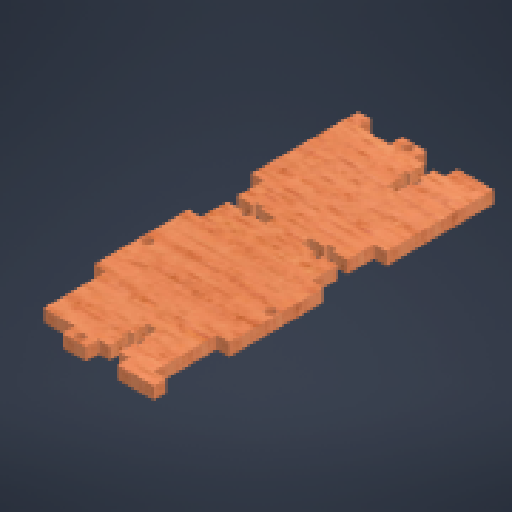
# Autodesk Inventor part: FloorButtonHolder_Top_V1
Saved by Autodesk Inventor 2024.1 (Build 281209000, 209)
## iProperties
Created: 2023-05-20
Part Number: FloorButtonHolder_Top_V1
Material: MDF Medium Density Fiberboard
Document SubType Name: Modeling
Designer: jaege
Density: 0.8 g/cm^3
Appearance: Red Oak - Natural Low Gloss
Author: jaege
Autodesk Inventor part; units mm, degrees
ref_plane "YZ Plane" through (0, 0, 0) normal (1, 0, 0) x (0, 1, 0)
ref_plane "XZ Plane" through (0, 0, 0) normal (0, 1, 0) x (-1, 0, 0)
ref_plane "XY Plane" through (0, 0, 0) normal (0, 0, 1) x (1, 0, 0)
sketch "Sketch1" plane through (0, 0, 0) normal (0, 1, 0) x (-1, 0, 0)
  line L0 (-17.5, 50) -> (17.5, 50)
  line L1 (17.5, 50) -> (17.5, -50)
  line L2 (17.5, -50) -> (-17.5, -50)
  line L3 (-17.5, -50) -> (-17.5, 50)
  line L4 (-17.5, 50) -> (17.5, -50) construction
  line L5 (17.5, 50) -> (-17.5, -50) construction
  line L6 (7.5, 50) -> (0, 50)
  line L7 (0, 50) -> (0, 54)
  line L8 (0, 54) -> (7.5, 54)
  line L9 (7.5, 54) -> (7.5, 50)
  line L10 (-10, 50) -> (-21.5, 50)
  line L11 (-21.5, 50) -> (-21.5, 54)
  line L12 (-21.5, 54) -> (-10, 54)
  line L13 (-10, 54) -> (-10, 50)
  line L14 (17.5, 30) -> (21.5, 30)
  line L15 (21.5, 30) -> (21.5, 0)
  line L16 (21.5, 0) -> (17.5, 0)
  line L17 (17.5, 0) -> (17.5, 30)
  line L18 (17.5, -20) -> (21.5, -20)
  line L19 (21.5, -20) -> (21.5, -54)
  line L20 (21.5, -54) -> (17.5, -54)
  line L21 (17.5, -54) -> (17.5, -20)
  line L22 (7.5, -50) -> (0, -50)
  line L23 (0, -50) -> (0, -54)
  line L24 (0, -54) -> (7.5, -54)
  line L25 (7.5, -54) -> (7.5, -50)
  line L26 (-10, -50) -> (-21.5, -50)
  line L27 (-21.5, -50) -> (-21.5, -54)
  line L28 (-21.5, -54) -> (-10, -54)
  line L29 (-10, -54) -> (-10, -50)
  line L30 (-17.5, 30) -> (-21.5, 30)
  line L31 (-21.5, 30) -> (-21.5, 0)
  line L32 (-21.5, 0) -> (-17.5, 0)
  line L33 (-17.5, 0) -> (-17.5, 30)
  line L34 (-17.5, -50) -> (-21.5, -50)
  line L35 (-21.5, -50) -> (-21.5, -20)
  line L36 (-21.5, -20) -> (-17.5, -20)
  line L37 (-17.5, -20) -> (-17.5, -50)
  point P0 (0, 0)
  point P1 (17.5, 0)
  point P2 (-17.5, 0)
  point P3 (-17.5, -20)
  point P4 (0, -50)
  point P5 (17.5, -50)
  dimension "d0" = 35
  dimension "d2" = 7.5
  dimension "d3" = 4
  dimension "d4" = 11.5
  dimension "d5" = 4
  dimension "d6" = 10
  dimension "d7" = 10
  dimension "d8" = 4
  dimension "d9" = 30
  dimension "d10" = 4
  dimension "d11" = 34
  dimension "d12" = 20
  dimension "d13" = 20
  dimension "d14" = 7.5
  dimension "d15" = 4
  dimension "d16" = 11.5
  dimension "d17" = 4
  dimension "d18" = 10
  dimension "d19" = 10
  dimension "d20" = 4
  dimension "d21" = 30
  dimension "d22" = 20
  dimension "d23" = 4
  dimension "d24" = 30
  dimension "d27" = 4
  constraints: 76 end point, 18 parallel, 9 horizontal, 9 perpendicular, 7 point on line, 2 midpoint
  measures "d0" distance of L1.end L2.end
  measures "d2" distance of L7.end L8.end
  measures "d3" distance of L6.end L7.end
  measures "d4" distance of L11.end L12.end
  measures "d5" distance of L10.end L11.end
  measures "d6" distance between parallel lines of L9 L1
  measures "d7" distance between parallel lines of L13 L7
  measures "d8" distance of L15.end L16.end
  measures "d9" distance of L14.end L15.end
  measures "d10" distance of L19.end L20.end
  measures "d11" distance of L18.end L19.end
  measures "d12" distance between parallel lines of L16 L18
  measures "d13" distance between parallel lines of L0 L14
  measures "d14" distance of L24.end L23.end
  measures "d15" distance of L23.end L22.end
  measures "d16" distance of L28.end L27.end
  measures "d17" distance of L27.end L26.end
  measures "d18" distance between parallel lines of L25 L21
  measures "d19" distance between parallel lines of L29 L23
  measures "d20" distance of L32.end L31.end
  measures "d21" distance of L31.end L30.end
  measures "d22" distance between parallel lines of L10 L30
  measures "d23" distance of L35.end L36.end
  measures "d24" distance of L34.end L35.end
  measures "d27" distance between parallel lines of L2 L20
extrude "Extrusion1" add sketch "Sketch1" along normal blind 4
sketch "Sketch3" plane through (0, 4, 0) normal (0, 1, 0) x (1, 0, 0)
  line L0 (17.5, 11.5) -> (5.5, 11.5)
  line L1 (5.5, 11.5) -> (5.5, 8.5)
  line L2 (5.5, 8.5) -> (17.5, 8.5)
  line L3 (17.5, 8.5) -> (17.5, 11.5)
  line L4 (10.3, 7.3) -> (12.7, 7.3)
  line L5 (12.7, 7.3) -> (12.7, 12.7)
  line L6 (12.7, 12.7) -> (10.3, 12.7)
  line L7 (10.3, 12.7) -> (10.3, 7.3)
  line L8 (17.5, 0) -> (17.5, 20) projected
  line L9 (10, -50) -> (0, -50) projected
  line L10 (3.5, -38) -> (6.5, -38)
  line L11 (6.5, -38) -> (6.5, -50)
  line L12 (6.5, -50) -> (3.5, -50)
  line L13 (3.5, -50) -> (3.5, -38)
  line L14 (2.3, -45.2) -> (7.7, -45.2)
  line L15 (7.7, -45.2) -> (7.7, -42.8)
  line L16 (7.7, -42.8) -> (2.3, -42.8)
  line L17 (2.3, -42.8) -> (2.3, -45.2)
  line L18 (-17.5, 11.5) -> (-5.5, 11.5)
  line L19 (-5.5, 11.5) -> (-5.5, 8.5)
  line L20 (-5.5, 8.5) -> (-17.5, 8.5)
  line L21 (-17.5, 8.5) -> (-17.5, 11.5)
  line L22 (-12.7, 7.3) -> (-10.3, 7.3)
  line L23 (-10.3, 7.3) -> (-10.3, 12.7)
  line L24 (-10.3, 12.7) -> (-12.7, 12.7)
  line L25 (-12.7, 12.7) -> (-12.7, 7.3)
  line L26 (0, -50) -> (10, -50) projected
  line L27 (-17.5, 20) -> (-17.5, 0) projected
  line L28 (3.5, 50) -> (6.5, 50)
  line L29 (6.5, 50) -> (6.5, 38)
  line L30 (6.5, 38) -> (3.5, 38)
  line L31 (3.5, 38) -> (3.5, 50)
  line L32 (10, 50) -> (0, 50) projected
  line L33 (2.3, 42.8) -> (7.7, 42.8)
  line L34 (7.7, 42.8) -> (7.7, 45.2)
  line L35 (7.7, 45.2) -> (2.3, 45.2)
  line L36 (2.3, 45.2) -> (2.3, 42.8)
  line L37 (10, 50) -> (0, 50) projected
  circle A0 centre (-19.5, -15) radius 1.5
  line L38 (0, 54) -> (-7.5, 54) projected
  line L39 (-7.5, 54) -> (0, 50) construction
  line L40 (-7.5, -54) -> (0, -54) projected
  line L41 (-7.5, -54) -> (0, -50) construction
  line L42 (-17.5, 0) -> (-21.5, 0) projected
  line L43 (-21.5, -30) -> (-17.5, 0) construction
  line L44 (21.5, 0) -> (17.5, 0) projected
  line L45 (17.5, 0) -> (21.5, -30) construction
  point P0 (0, 0)
  point P1 (11.5, 12.7)
  point P2 (11.5, 8.5)
  point P3 (12.7, 10)
  point P4 (17.5, 10)
  point P5 (17.5, 10)
  point P6 (2.3, -44)
  point P7 (6.5, -44)
  point P8 (5, -42.8)
  point P9 (5, -38)
  point P10 (-12.7, 10)
  point P11 (-5.5, 10)
  point P12 (-11.5, 12.7)
  point P13 (-11.5, 11.5)
  point P14 (5, -50)
  point P15 (5, -50)
  point P16 (5, -50)
  point P17 (-17.5, 10)
  point P18 (5, 38)
  point P19 (5, 50)
  point P20 (5, 50)
  point P21 (2.3, 44)
  point P22 (3.5, 44)
  point P23 (5, 45.2)
  point P24 (5, 50)
  point P25 (10.3, 11.5)
  point P26 (10.3, 8.5)
  point P27 (12.7, 8.5)
  point P28 (12.7, 11.5)
  point P29 (6.5, 45.2)
  point P30 (3.5, 45.2)
  point P31 (3.5, 42.8)
  point P32 (6.5, 42.8)
  point P33 (6.5, -42.8)
  point P34 (3.5, -42.8)
  point P35 (3.5, -45.2)
  point P36 (6.5, -45.2)
  point P37 (-10.3, 8.5)
  point P38 (-10.3, 11.5)
  point P39 (-12.7, 11.5)
  point P40 (-12.7, 8.5)
  dimension "d35" = 12
  dimension "d36" = 3
  dimension "d37" = 2.4
  dimension "d38" = 5.4
  dimension "d39" = 3
  dimension "d40" = 12
  dimension "d41" = 5.4
  dimension "d42" = 2.4
  dimension "d43" = 12
  dimension "d44" = 3
  dimension "d45" = 2.4
  dimension "d46" = 5.4
  dimension "d47" = 3
  dimension "d51" = 12
  dimension "d52" = 2.4
  dimension "d53" = 5.4
  dimension "d54" = 3
  constraints: 72 end point, 25 midpoint, 16 parallel, 8 horizontal, 8 perpendicular, 7 horizontal alignment, 6 vertical alignment, 4 coincident, 1 centre point, 1 other
  measures "d35" distance of L2.end L1.end
  measures "d36" distance of L1.end L0.end
  measures "d37" distance of L6.end L5.end
  measures "d38" distance of L5.end L4.end
  measures "d39" distance of L11.end L12.end
  measures "d40" distance of L10.end L11.end
  measures "d41" distance of L16.end L15.end
  measures "d42" distance of L15.end L14.end
  measures "d43" distance of L19.end L21.start
  measures "d44" distance of L18.end L19.end
  measures "d45" distance of L24.end L24.start
  measures "d46" distance of L24.start L23.start
  measures "d47" distance of L29.end L30.end
  measures "d51" distance of L28.end L29.end
  measures "d52" distance of L35.end L33.start
  measures "d53" distance of L33.start L33.end
  measures "d54" diameter of A0
extrude "Extrusion3" cut sketch "Sketch3" against normal up to next
body "Solid1"
